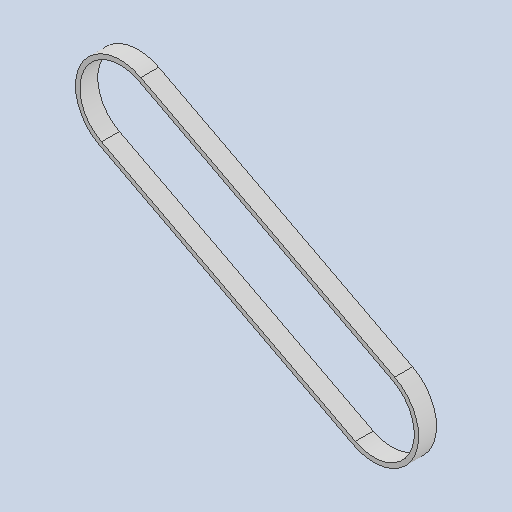
# Autodesk Inventor part: Lift up banding
Saved by Autodesk Inventor 2022.2 (Build 262287010, 287A)
## iProperties
Created: 2022-06-29
Part Number: Lift up banding
Material: Generic
Document SubType Name: Modeling
Designer: Main Account
Density: 1 g/cm^3
Appearance: Default
Author: Main Account
Autodesk Inventor part; units mm, degrees
ref_plane "YZ Plane" through (0, 0, 0) normal (1, 0, 0) x (0, 1, 0)
ref_plane "XZ Plane" through (0, 0, 0) normal (0, 1, 0) x (-1, 0, 0)
ref_plane "XY Plane" through (0, 0, 0) normal (0, 0, 1) x (1, 0, 0)
sketch "Sketch1" plane through (0, 0, 0) normal (0, 0, 1) x (1, 0, 0)
  circle A0 centre (-72.1123, 37.6359) radius 14.0335 construction
  arc A1 (-5.2885, -10.133) -> (5.2885, 10.133) centre (0, 0) ccw
  arc A2 (-5.8761, -11.2589) -> (5.8761, 11.2589) centre (0, 0) ccw
  arc A3 (-66.8239, 47.7689) -> (-77.4008, 27.503) centre (-72.1123, 37.6359) ccw
  arc A4 (-66.2362, 48.8948) -> (-77.9884, 26.3771) centre (-72.1123, 37.6359) ccw
  line L0 (-5.8761, -11.2589) -> (-77.9884, 26.3771)
  line L1 (5.8761, 11.2589) -> (-66.2362, 48.8948)
  line L2 (-66.8239, 47.7689) -> (5.2885, 10.133)
  line L3 (-5.2885, -10.133) -> (-77.4008, 27.503)
  dimension "d0" = 22.86
  dimension "d1" = 25.4
  dimension "d2" = 22.86
  dimension "d3" = 25.4
  constraints: 8 end point, 8 point on circle, 6 tangent, 4 centre point, 4 coincident, 2 parallel
  measures "d0" diameter of A1
  measures "d1" diameter of A2
  measures "d2" diameter of A3
  measures "d3" diameter of A4
extrude "Extrusion1" add sketch "Sketch1" against normal blind 5.08
body "Solid1"
